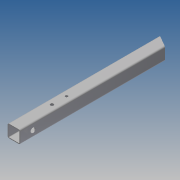
# Autodesk Inventor part: 2f2ax1
Saved by Autodesk Inventor 2014 SP1 (Build 180222100, 222)
## iProperties
Company: HERA Project
Created: 2013-06-27
Part Number: 2f2ax1
Material: Steel
Description: Feed backplane support interior piece
Document SubType Name: Modeling
Designer: David DeBoer
Mass: 156.218 g
Surface Area: 246.159 cm^2
Volume: 19.9004 cm^3
Density: 7.85 g/cm^3
Appearance: Steel
Title: Feed backplane support interior piece
Author: David DeBoer
Autodesk Inventor part; units mm, degrees
ref_plane "YZ Plane" through (0, 0, 0) normal (1, 0, 0) x (0, 1, 0)
ref_plane "XZ Plane" through (0, 0, 0) normal (0, 1, 0) x (-1, 0, 0)
ref_plane "XY Plane" through (0, 0, 0) normal (0, 0, 1) x (1, 0, 0)
sketch "Sketch1" plane through (0, 0, 0) normal (0, 0, 1) x (1, 0, 0)
  line L0 (3.7363, 0) -> (22.7863, 0)
  line L1 (25.9613, 3.175) -> (25.9613, 22.225)
  line L2 (22.7863, 25.4) -> (3.7363, 25.4)
  line L3 (0.5613, 22.225) -> (0.5613, 3.175)
  arc A0 (3.7363, 25.4) -> (0.5613, 22.225) centre (3.7363, 22.225) ccw
  arc A1 (0.5613, 3.175) -> (3.7363, 0) centre (3.7363, 3.175) ccw
  arc A2 (22.7863, 0) -> (25.9613, 3.175) centre (22.7863, 3.175) ccw
  arc A3 (25.9613, 22.225) -> (22.7863, 25.4) centre (22.7863, 22.225) ccw
  line L4 (3.7363, 23.749) -> (22.7863, 23.749)
  arc A4 (24.3103, 22.225) -> (22.7863, 23.749) centre (22.7863, 22.225) ccw
  line L5 (24.3103, 22.225) -> (24.3103, 3.175)
  arc A5 (22.7863, 1.651) -> (24.3103, 3.175) centre (22.7863, 3.175) ccw
  line L6 (22.7863, 1.651) -> (3.7363, 1.651)
  arc A6 (2.2123, 3.175) -> (3.7363, 1.651) centre (3.7363, 3.175) ccw
  line L7 (2.2123, 3.175) -> (2.2123, 22.225)
  arc A7 (3.7363, 23.749) -> (2.2123, 22.225) centre (3.7363, 22.225) ccw
  point P0 (0, 0)
  point P1 (0.5613, 0)
  point P2 (25.9613, 0)
  point P3 (0.5613, 25.4)
  dimension "d0" = 25.4
  dimension "d2" = 25.4
  dimension "d3" = 3.175
  dimension "d4" = 1.651
  constraints: 16 end point, 16 point on circle, 8 centre point, 8 tangent, 6 point on line, 4 parallel, 3 equal radius, 2 perpendicular, 1 horizontal, 7 other
  measures "d0" distance of point (0.561, 0) point (25.961, 0)
  measures "d2" distance of point (0.561, 25.4) point (0.561, 0)
  measures "d3" radius of A0
  measures "d4" distance between parallel lines of L4 L2
extrude "Extrusion1" add sketch "Sketch1" along normal blind 304.8
sketch "Sketch2" plane through (3.7363, 25.4, 0) normal (0, 1, 0) x (1, 0, 0)
  line L0 (22.2338, 0) -> (22.2338, -14.667)
  line L1 (22.2338, 0) -> (-3.1718, 0)
  line L2 (-3.1718, 0) -> (22.2338, -14.667)
  point P0 (-3.7363, 0)
  constraints: 6 end point, 1 perpendicular
extrude "Extrusion2" cut sketch "Sketch2" against normal blind 149.86
sketch "Sketch3" plane through (3.7363, 25.4, 304.8) normal (0, 1, 0) x (1, 0, 0)
  line L0 (19.05, 291.9711) -> (0, 302.9689) projected
  line L1 (0, 302.9689) -> (0, 0) projected
  line L2 (19.05, 0) -> (0, 0) projected
  line L3 (19.05, 291.9711) -> (19.05, 0) projected
  line L4 (9.525, 0) -> (9.525, 297.47) construction
  point P0 (-3.7363, 304.8)
  constraints: 2 end point, 2 midpoint, 1 parallel
sketch "Sketch4" plane through (3.7363, 25.4, 304.8) normal (0, 1, 0) x (1, 0, 0)
  line L0 (19.05, 291.9711) -> (0, 302.9689) projected
  line L1 (19.05, 0) -> (0, 0) projected
  line L2 (9.525, 0) -> (9.525, 297.47) construction
  circle A0 centre (9.525, 76.2) radius 2.9006
  point P0 (-3.7363, 304.8)
  dimension "d11" = 76.2
  constraints: 2 end point, 2 midpoint, 1 centre point, 1 point on line
  measures "d11" distance from line of A0.centre L1
hole "Hole1" at (13.2613, 25.4, 228.6) direction (0, -1, 0) diameter 6.35 end through all
sketch "Sketch5" plane through (3.7363, 0, 304.8) normal (0, -1, 0) x (1, 0, 0)
  circle A0 centre (9.525, -76.2) radius 3.175 projected
  circle A1 centre (9.525, -111.76) radius 2.1428
  point P0 (-3.7363, -304.8)
  dimension "d19" = 35.56
  constraints: 1 centre point
  measures "d19" distance of A1.centre A0.centre
hole "Hole2" at (13.2613, 0, 193.04) direction (0, 1, 0) diameter 3.9624 depth 16.51 tip angle 118 thread size "10-32 UNF" class "2B" standard "ANSI Unified Screw Threads"
sketch "Sketch6" plane through (25.9613, 3.175, 304.8) normal (1, 0, 0) x (0, 0, -1)
  line L0 (0, 0) -> (0, 19.05) projected
  circle A0 centre (25.4, 9.525) radius 2.9685
  point P0 (304.8, -3.175)
  dimension "d27" = 25.4
  constraints: 1 centre point
  measures "d27" distance from line of A0.centre L0
hole "Hole3" at (25.9613, 12.7, 279.4) direction (-1, 0, 0) diameter 9.525 end through all
sketch "Sketch7" plane through (3.7363, 25.4, 304.8) normal (0, 1, 0) x (1, 0, 0)
  circle A0 centre (9.525, 76.2) radius 3.175 projected
  circle A1 centre (9.525, 105.41) radius 3.5498
  point P0 (-3.7363, 304.8)
  dimension "d35" = 29.21
  constraints: 1 centre point
  measures "d35" distance of A1.centre A0.centre
hole "Hole4" at (13.2613, 25.4, 199.39) direction (0, -1, 0) diameter 5.1054 depth 25.4 tip angle 118 clearance for "Flat Head Machine Screw (82)" size "#10" standard "Ansi Unified Screw Threads"
body "Solid1"
